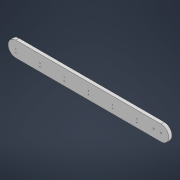
# Autodesk Inventor part: Motor linkage
Saved by Autodesk Inventor 2021 (Build 250183000, 183)
## iProperties
Created: 2021-04-18
Part Number: Motor linkage
Material: Generic
Document SubType Name: Modeling
Designer: allen
Density: 1 g/cm^3
Appearance: Default
Author: allen
Autodesk Inventor part; units mm, degrees
ref_plane "YZ Plane" through (0, 0, 0) normal (1, 0, 0) x (0, 1, 0)
ref_plane "XY Plane" through (0, 0, 0) normal (0, 0, 1) x (1, 0, 0)
sketch "Sketch1" plane through (0, 0, 0) normal (0, 0, 1) x (1, 0, 0)
  line L0 (112.5, 0) -> (-112.5, 0) construction
  line L1 (112.5, 12) -> (-112.5, 12)
  line L2 (-112.5, -12) -> (112.5, -12)
  arc A0 (112.5, -12) -> (112.5, 12) centre (112.5, 0) ccw
  arc A1 (-112.5, 12) -> (-112.5, -12) centre (-112.5, 0) ccw
  point P0 (0, 0)
  dimension "d0" = 225
  dimension "d1" = 12
  constraints: 8 end point, 4 point on circle, 4 tangent, 2 centre point, 1 horizontal, 1 midpoint, 1 parallel
  measures "d0" distance of L0.start L0.end
  measures "d1" radius of A0
extrude "Extrusion1" add sketch "Sketch1" along normal blind 5
sketch "Sketch2" plane through (0, 0, 5) normal (0, 0, 1) x (1, 0, 0)
  arc A0 (112.5, -12) -> (112.5, 12) centre (112.5, 0) ccw projected
  point P0 (0, 0)
  constraints: 1 coincident
hole "Hole1" at (112.5, 0, 5) direction (0, 0, -1) diameter 1.9 end through all
sketch "Sketch3" plane through (0, 0, 5) normal (0, 0, 1) x (1, 0, 0)
  arc A0 (-112.5, 12) -> (-112.5, -12) centre (-112.5, 0) ccw projected
  circle A1 centre (112.5, 0) radius 0.95 projected
  point P0 (0, 0)
  point P1 (75, 0)
  point P2 (37.5, 0)
  point P3 (0, 0)
  point P4 (-37.5, 0)
  point P5 (-75, 0)
  dimension "d33" = 37.5
  dimension "d34" = 37.5
  dimension "d35" = 37.5
  dimension "d36" = 37.5
  constraints: 4 horizontal alignment, 2 coincident
  measures "d33" distance of A1.centre point (75, 0)
  measures "d34" distance of point (37.5, 0) point (75, 0)
  measures "d35" distance of point (0, 0) point (-37.5, 0)
  measures "d36" distance of point (-37.5, 0) point (-75, 0)
hole "Hole2" at (-112.5, 0, 5) at (-75, 0, 5) at (-37.5, 0, 5) at (0, 0, 5) at (37.5, 0, 5) at (75, 0, 5) direction (0, 0, -1) diameter 1 end through all
sketch "Sketch4" plane through (0, 0, 5) normal (0, 0, 1) x (1, 0, 0)
  circle A0 centre (112.5, 0) radius 0.95 projected
  point P0 (0, 0)
  point P1 (105, 0)
  point P2 (101.15, 0)
  dimension "d18" = 7.5
  dimension "d32" = 3.85
  constraints: 2 horizontal alignment
  measures "d18" distance of A0.centre point (105, 0)
  measures "d32" distance of point (105, 0) point (101.15, 0)
hole "Hole3" at (101.15, 0, 5) direction (0, 0, -1) diameter 1.8 end through all
ref_plane "Work Plane1" through (0, -2.5, 0) normal (0, 1, 0) x (-1, 0, 0)
mirror "Mirror1" about plane through (0, -2.5, 0) normal (0, 1, 0) of "Hole2"
sketch "Sketch5" plane through (0, 0, 5) normal (0, 0, 1) x (1, 0, 0)
  circle A0 centre (112.5, 0) radius 0.95 projected
  point P0 (0, 0)
equation "\"d34\" = d33"
equation "\"d35\" = d34"
equation "\"d36\" = d35"
body "Solid1"
